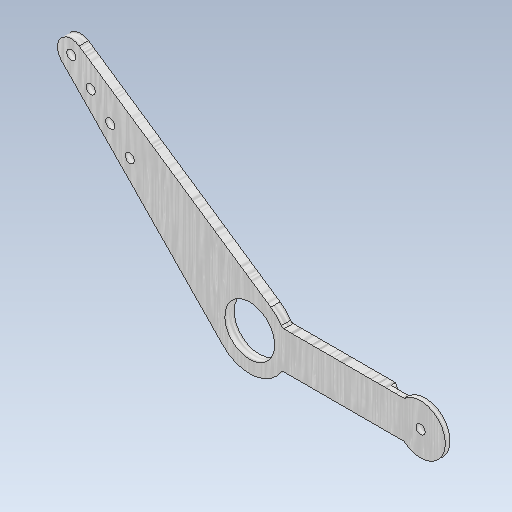
# Autodesk Inventor part: アーム中間その弐
Saved by Autodesk Inventor 2020.2 (Build 242310000, 310)
## iProperties
Created: 2020-02-28
Part Number: アーム中間その弐
Material: アルミニウム 7075
Document SubType Name: Modeling
Designer: aoyam
Density: 2.81 g/cm^3
Appearance: サテン - ブラシ仕上げ 重厚
Mass: 12.7298 g
Surface Area: 52.803 cm^2
Volume: 4.53019 cm^3
Author: aoyam
Autodesk Inventor part; units mm, degrees
ref_plane "YZ Plane" through (0, 0, 0) normal (1, 0, 0) x (0, 1, 0)
ref_plane "XZ Plane" through (0, 0, 0) normal (0, 1, 0) x (-1, 0, 0)
ref_plane "XY Plane" through (0, 0, 0) normal (0, 0, 1) x (1, 0, 0)
sketch "スケッチ1" plane through (0, 0, 0) normal (0, 0, 1) x (1, 0, 0)
  circle A0 centre (-55, 0) radius 8.025
  circle A1 centre (-55, 0) radius 12.025
  line L0 (6, -6) -> (-61, -6)
  line L1 (-61, -6) -> (-61, 6)
  line L2 (-61, 6) -> (6, 6)
  line L3 (-61, -6) -> (-61, 6)
  line L4 (-20.8557, 4.9841) -> (202.5072, 4.9841) construction
  circle A2 centre (0, 0) radius 8
  line L5 (-23.9175, 26.3005) -> (3.7655, 4.6721)
  circle A3 centre (0, 0) radius 1.5
  circle A4 centre (0, 0) radius 3
  line L6 (-23.8151, -6) -> (-9.3095, 2.3748)
  line L7 (-9.3095, 2.3748) -> (-11, 6)
  line L8 (-55, 0) -> (0, 0)
  line L9 (0, 0) -> (0, 6)
  line L10 (-55, 0) -> (-112.4533, 48.2091)
  circle A5 centre (-112.4533, 48.2091) radius 4.5
  line L11 (-48.2337, 9.9407) -> (-109.9213, 51.9291)
  line L12 (-115.6772, 45.0695) -> (-63.6148, -8.3897)
  circle A6 centre (-112.4533, 48.2091) radius 1.5
  line L13 (-112.4533, 48.2091) -> (-74.1421, 8.87)
  circle A7 centre (-106.1742, 41.7614) radius 1.5
  circle A8 centre (-99.895, 35.3138) radius 1.5
  circle A9 centre (-93.6158, 28.8662) radius 1.5
  circle A10 centre (-57.5782, 13.277) radius 1.5
  circle A11 centre (-55, 0) radius 11 construction
  circle A12 centre (-57.5782, 13.277) radius 2.5
  point P0 (-62.7295, -9.2117)
  point P1 (-47.2705, 9.2117)
  point P2 (-5.2915, 6)
  point P3 (-5.2915, -6)
  point P4 (-44.5788, 6)
  point P5 (-44.5788, -6)
  point P6 (-49.6708, 6)
  point P7 (-49.6708, -6)
  point P8 (-60.3292, -6)
  point P9 (-61, -5.3292)
  point P10 (-61, 5.3292)
  point P11 (-60.3292, 6)
  point P12 (2.066, 6)
  point P13 (5.2915, -6)
  point P14 (5.2915, 6)
  point P15 (-57.2923, 11.8045)
  point P16 (-56.1715, 15.3437)
  point P17 (-55.4185, 12.0177)
  point P18 (-59.1096, 11.301)
  dimension "d1" = 16.05
  dimension "d3" = 4
  dimension "d19" = 38
  dimension "d35" = 16
  dimension "d36" = 3
  dimension "d37" = 6
  dimension "d38" = 55
  dimension "d39" = 6
  dimension "d40" = 6
  dimension "d42" = 65
  dimension "d43" = 11
  dimension "d44" = 4
  dimension "d45" = 30
  dimension "d47" = 75
  dimension "d50" = 9
  dimension "d51" = 3
  dimension "d54" = 9
  dimension "d59" = 140
  dimension "d63" = 9
  dimension "d67" = 3
  dimension "d68" = 22
  dimension "d69" = 1
  constraints: 28 end point, 13 centre point, 6 coincident, 6 point on circle, 6 tangent, 3 horizontal, 3 point on line, 2 parallel, 2 perpendicular, 8 other
  measures "d1" diameter of A0
  measures "d3" radial gap between concentric circles of A0 A1
  measures "d19" angle of L2 L5
  measures "d35" diameter of A2
  measures "d36" diameter of A3
  measures "d37" diameter of A4
  measures "d38" distance of L8.start L8.end
  measures "d39" distance between parallel lines of L8 L0
  measures "d40" distance between parallel lines of L2 L8
  measures "d42" angle of L2 L7
  measures "d43" distance from line of L7.end L9
  measures "d44" distance of L6.end L7.end
  measures "d45" angle of L6 L0
  measures "d47" distance of L8.start L10.end
  measures "d50" diameter of A5
  measures "d51" diameter of A6
  measures "d54" distance of L13.start A7.centre
  measures "d59" angle of L8 L10
  measures "d63" distance of A7.centre L10.end
  measures "d67" diameter of A10
  measures "d68" diameter of A11
  measures "d69" radial gap between concentric circles of A10 A12
extrude "押し出し1" add sketch "スケッチ1" along normal blind 3 contours L8 A1 L0 A0 | A0 L2 A1 L8 | A0 L2 L1 L10 A1 A12 | L0 A1 L10 A0 L1 | L8 L6 L0 A1 | A1 L2 L7 L6 L8 | A0 L1 L2 | L0 L1 A0 | L8 A2 L0 L6 | L6 L7 L2 A2 L8 | A1 A12 L11 | L12 A5 L13 A7 L10 A1 | L8 A4 L9 L2 A2 L0 | A2 L2 L9 A4 L8 | A12 A1 | A10 | A1 A12 | A12 A1 L10 A7 A5 L11 | A2 L5 L2 | A5 L10 A6 L13 | L0 A2 | L8 A3 L9 A4 | A4 L9 A3 L8 | A2 L2 L5 | L13 A6 L10 A5 | A5 L10 A7 L13
extrude "押し出し3" cut sketch "スケッチ1" along normal blind 1.5 contours L8 A2 L0 L6 | L6 L7 L2 A2 L8 | L8 A4 L9 L2 A2 L0 | A2 L2 L9 A4 L8 | A2 L5 L2 | L0 A2 | A2 L2 L5
sketch "スケッチ2" plane through (0, 0, 3) normal (0, 0, 1) x (1, 0, 0)
  circle A0 centre (-55, 0) radius 8.025 projected
  circle A1 centre (0, 0) radius 1.5 projected
  arc A2 (-44.5788, 6) -> (-48.2337, 9.9407) centre (-55, 0) ccw projected
  line L0 (-48.2337, 9.9407) -> (-109.9213, 51.9291) projected
  arc A3 (-109.9213, 51.9291) -> (-115.6772, 45.0695) centre (-112.4533, 48.2091) ccw projected
  line L1 (-115.6772, 45.0695) -> (-63.6148, -8.3897) projected
  arc A4 (-63.6148, -8.3897) -> (-44.5788, -6) centre (-55, 0) ccw projected
  line L2 (-44.5788, -6) -> (-5.2915, -6) projected
  arc A5 (-5.2915, -6) -> (-5.2915, 6) centre (0, 0) ccw projected
  line L3 (-5.2915, 6) -> (-44.5788, 6) projected
  circle A6 centre (-112.4533, 48.2091) radius 1.5 projected
  circle A7 centre (-93.6158, 28.8662) radius 1.5 projected
  circle A8 centre (-99.895, 35.3138) radius 1.5 projected
  circle A9 centre (-106.1742, 41.7614) radius 1.5 projected
  dimension "d64" = 9
  dimension "d65" = 9
  dimension "d66" = 9
  measures "d64" distance of A9.centre A3.centre
  measures "d65" distance of A8.centre A9.centre
  measures "d66" distance of A7.centre A8.centre
sketch "スケッチ3" plane through (0, 0, 0) normal (0, 0, -1) x (-1, 0, 0)
  circle A0 centre (106.1742, 41.7614) radius 1.5 projected
  circle A1 centre (99.895, 35.3138) radius 1.5 projected
  circle A2 centre (93.6158, 28.8662) radius 1.5 projected
  circle A3 centre (112.4533, 48.2091) radius 1.5 projected
  line L0 (11, 6) -> (9.3095, 2.3748) projected
  line L1 (9.3095, 2.3748) -> (23.8151, -6) projected
  line L2 (44.5788, -6) -> (23.8151, -6) projected
  arc A4 (44.5788, -6) -> (63.6148, -8.3897) centre (55, 0) ccw projected
  line L3 (115.6772, 45.0695) -> (63.6148, -8.3897) projected
  arc A5 (115.6772, 45.0695) -> (109.9213, 51.9291) centre (112.4533, 48.2091) ccw projected
  line L4 (48.2337, 9.9407) -> (109.9213, 51.9291) projected
  arc A6 (48.2337, 9.9407) -> (44.5788, 6) centre (55, 0) ccw projected
  line L5 (11, 6) -> (44.5788, 6) projected
  circle A7 centre (55, 0) radius 8.025 projected
  arc A8 (78.5193, -24.8633) -> (80.7612, -22.8663) centre (79.3836, -23.5767) ccw
  line L6 (78.5193, -24.8633) -> (60.9226, -13.0433)
  arc A9 (61.0119, -10.4143) -> (60.9226, -13.0433) centre (61.7868, -11.7567) ccw
  arc A10 (61.0119, -10.4143) -> (66.3, -4.1122) centre (55, 0) ccw
  arc A11 (68.8736, -3.5676) -> (66.3, -4.1122) centre (67.7566, -4.6422) ccw
  line L7 (68.8736, -3.5676) -> (80.9904, -16.1632)
  arc A12 (81.1255, -18.1514) -> (80.9904, -16.1632) centre (79.8733, -17.2378) ccw
  arc A13 (81.1255, -18.1514) -> (80.7612, -22.8663) centre (84.7607, -20.8038) ccw
  arc A14 (40.2559, -2) -> (40.2559, 2) centre (40.2559, 0) ccw
  line L8 (40.2559, -2) -> (22.4227, -2)
  arc A15 (22.4227, 2) -> (22.4227, -2) centre (22.4227, 0) ccw
  line L9 (22.4227, 2) -> (40.2559, 2)
  line L10 (9.3095, -2.3748) -> (11, -6)
  line L11 (44.5788, -6) -> (11, -6)
  arc A16 (44.5788, -6) -> (48.2949, -9.9821) centre (55, 0) ccw
  line L12 (102.7709, -46.5745) -> (48.2949, -9.9821)
  arc A17 (102.7709, -46.5745) -> (109.1623, -38.9576) centre (105.5589, -42.424) ccw
  line L13 (63.6661, 8.3366) -> (109.1623, -38.9576)
  arc A18 (63.6661, 8.3366) -> (44.5788, 6) centre (55, 0) ccw
  line L14 (23.8151, 6) -> (44.5788, 6)
  line L15 (23.8151, 6) -> (9.3095, -2.3748)
  circle A19 centre (55, 0) radius 8.025
  circle A20 centre (84.7607, -20.8038) radius 1.5
  circle A21 centre (105.5589, -42.424) radius 1.5
  circle A22 centre (91.6934, -28.0105) radius 1.5
  circle A23 centre (98.6262, -35.2172) radius 1.5
  line L16 (55, 0) -> (46.975, 0)
  arc A24 (80.7612, 22.8663) -> (78.5193, 24.8633) centre (79.3836, 23.5767) ccw
  line L17 (78.5193, 24.8633) -> (60.9226, 13.0433)
  arc A25 (60.9226, 13.0433) -> (61.0119, 10.4143) centre (61.7868, 11.7567) ccw
  arc A26 (66.3, 4.1122) -> (61.0119, 10.4143) centre (55, 0) ccw
  arc A27 (66.3, 4.1122) -> (68.8736, 3.5676) centre (67.7566, 4.6422) ccw
  line L18 (68.8736, 3.5676) -> (80.9904, 16.1632)
  arc A28 (80.9904, 16.1632) -> (81.1255, 18.1514) centre (79.8733, 17.2378) ccw
  arc A29 (80.7612, 22.8663) -> (81.1255, 18.1514) centre (84.7607, 20.8038) ccw
  arc A30 (40.2559, -2) -> (40.2559, 2) centre (40.2559, 0) ccw
  line L19 (40.2559, 2) -> (22.4227, 2)
  arc A31 (22.4227, 2) -> (22.4227, -2) centre (22.4227, 0) ccw
  line L20 (22.4227, -2) -> (40.2559, -2)
  point P0 (0, 0)
  point P1 (0, 0)
  point P2 (61.0119, 10.4143)
  constraints: 38 point on circle, 30 end point, 23 centre point, 17 symmetric about line, 1 horizontal alignment, 10 other
extrude "押し出し4" cut sketch "スケッチ3" against normal blind 2.5 contours A25 L17 A24 A29 A28 L18 A27 L13 A18 | L13 A27 A26 | L8 A15 L9 A14
fillet "フィレット2" radius 1 2 edges at (-44.5788, 6, 1.5) (-44.5788, -6, 1.5)
